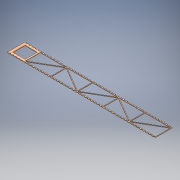
# Autodesk Inventor part: bottom
Saved by Autodesk Inventor 2018.3 (Build 223284000, 284)
## iProperties
Created: 2018-05-24
Part Number: bottom
Material: Wood (Birch)
Document SubType Name: Modeling
Designer: mzhang
Density: 0.55 g/cm^3
Appearance: Birch - Natural Polished
Mass: 4.54021 g
Surface Area: 164.361 cm^2
Volume: 8.25494 cm^3
Author: mzhang
Autodesk Inventor part; units mm, degrees
ref_plane "YZ Plane" through (0, 0, 0) normal (1, 0, 0) x (0, 1, 0)
ref_plane "XZ Plane" through (0, 0, 0) normal (0, 1, 0) x (-1, 0, 0)
ref_plane "XY Plane" through (0, 0, 0) normal (0, 0, 1) x (1, 0, 0)
sketch "Sketch1" plane through (0, 0, 0) normal (0, 0, 1) x (1, 0, 0)
  line L0 (0, 0) -> (40, 0)
  line L1 (40, 0) -> (40, 40)
  line L2 (40, 40) -> (0, 40)
  line L3 (0, 40) -> (0, 0)
  line L4 (45, 40) -> (45, -3.586)
  line L5 (470, 43.586) -> (470, -5)
  line L6 (472.0842, 45.0353) -> (472.0575, -4.9647)
  line L7 (45, 40) -> (45, -3.586)
  line L8 (470, -5) -> (470, 43.586)
  line L9 (45, -3.586) -> (128.586, 45)
  line L10 (46.414, -5) -> (129.078, 43.0501)
  line L11 (129.078, -5) -> (129.078, 43.0501)
  line L12 (131, 43.0501) -> (131, -5)
  line L13 (131, -5) -> (129, 45) construction
  line L14 (129.078, -5) -> (131.078, 45) construction
  line L15 (214, -3.0047) -> (214, 45)
  line L16 (216, 45) -> (216, -3.0047)
  line L17 (299.078, -5) -> (299.078, 43.0501)
  line L18 (301, 43.0501) -> (301, -5)
  line L19 (301, -5) -> (299, 45) construction
  line L20 (299.078, -5) -> (301.078, 45) construction
  line L21 (384.0797, -3.0079) -> (384.0797, 44.9968)
  line L22 (386, 45) -> (386, -3.0501)
  line L23 (386.0782, -5.0063) -> (384.0797, 44.9968) construction
  line L24 (384, -5) -> (386, 45) construction
  line L25 (214, -3.0047) -> (131.414, 45)
  line L26 (213.664, -5) -> (131, 43.0501)
  line L27 (216.414, -5) -> (299.078, 43.0501)
  line L28 (216, -3.0047) -> (298.586, 45)
  line L29 (384.0797, -3.0079) -> (301.4937, 44.9968)
  line L30 (383.664, -5) -> (301, 43.0501)
  line L31 (386, -3.0501) -> (468.586, 45)
  line L32 (386.414, -5) -> (469.078, 43.0501)
  line L33 (469.078, 43.0501) -> (470, 43.586)
  line L34 (-7, 45) -> (40, 45)
  line L35 (0, 45) -> (9, 45)
  line L36 (-7, 45) -> (-7, -5)
  line L37 (-7, -5) -> (40, -5)
  line L38 (40, 45) -> (45, 45)
  line L39 (45, 45) -> (45, 40)
  line L40 (-8.9425, 47.0353) -> (-8.9425, -6.9647)
  line L41 (472.0575, 47.0353) -> (472.0842, 47.0353)
  line L42 (472.0842, 47.0353) -> (472.0842, 45.0353)
  line L43 (472.0575, -4.9647) -> (472.0575, -6.9647)
  line L44 (-8.9425, 47.0353) -> (472.0842, 47.0353)
  line L45 (472.0575, -6.9647) -> (-8.9425, -6.9647)
  line L46 (45, 45) -> (128.586, 45)
  line L47 (131.414, 45) -> (214, 45)
  line L48 (216, 45) -> (298.586, 45)
  line L49 (301.4937, 44.9968) -> (384.0797, 44.9968)
  line L50 (386, 45) -> (468.586, 45)
  line L51 (213.664, -5) -> (131, -5)
  line L52 (40, -5) -> (129.078, -5)
  line L53 (216.414, -5) -> (299.078, -5)
  line L54 (301, -5) -> (383.664, -5)
  line L55 (386.414, -5) -> (470, -5)
  point P0 (20, 20)
  point P1 (385, -3.586)
  point P2 (215, -3.586)
  dimension "d0" = 40
  dimension "d1" = 40
  constraints: 113 end point, 12 parallel, 11 point on line, 6 perpendicular, 4 collinear, 4 horizontal, 2 vertical
  measures "d0" distance of L2.end L1.end
  measures "d1" distance of L1.end L0.end
extrude "Extrusion1" add sketch "Sketch1" along normal blind 1.5875
sketch "Sketch2" plane through (-8.9425, -6.9647, 0) normal (0, -1, 0) x (1, 0, 0)
  line L0 (0, 0) -> (0, 1.5875) projected
  line L1 (481.0267, 1.5875) -> (0, 1.5875) projected
  line L2 (0, 0) -> (5, 0)
  line L3 (5, 0) -> (5, 1.5875)
  line L4 (5, 1.5875) -> (0, 1.5875)
  line L5 (0, 1.5875) -> (0, 0)
  point P0 (8.9425, 0)
  dimension "d64" = 5
  constraints: 8 end point, 2 parallel, 1 horizontal, 1 perpendicular, 1 point on line
  measures "d64" distance of L4.end L3.end
extrude "Extrusion2" add sketch "Sketch2" along normal blind 1.5875
pattern_linear "Rectangular Pattern1" count 48 spacing 10 along (1, 0, 0) of "Extrusion2"
sketch "Sketch3" plane through (-8.9425, 47.0353, 0) normal (0, 1, 0) x (1, 0, 0)
  line L0 (0, 0) -> (481.0267, 0) projected
  line L1 (481.0267, -1.5875) -> (0, -1.5875) projected
  line L2 (0, 0) -> (5, 0)
  line L3 (5, 0) -> (5, -1.5875)
  line L4 (5, -1.5875) -> (0, -1.5875)
  line L5 (0, -1.5875) -> (0, 0)
  point P0 (8.9425, 0)
  dimension "d70" = 5
  constraints: 8 end point, 2 parallel, 1 horizontal, 1 perpendicular, 1 point on line
  measures "d70" distance of L3.end L4.end
extrude "Extrusion3" add sketch "Sketch3" along normal blind 1.5875
pattern_linear "Rectangular Pattern2" count 48 spacing 10 along (1, 0, 0) of "Extrusion3"
sketch "Sketch4" plane through (0, 0, 1.5875) normal (0, 0, 1) x (1, 0, 0)
  line L0 (472.0575, -6.9647) -> (472.0575, -4.9647) projected
  line L1 (472.0575, -6.9647) -> (473.7973, -6.9647)
  line L2 (473.7973, -6.9647) -> (473.7973, 49.231)
  line L3 (473.7973, 49.231) -> (472.0575, 49.231)
  line L4 (472.0575, 49.231) -> (472.0575, -6.9647)
  point P0 (0, 0)
  constraints: 8 end point, 2 parallel, 1 horizontal, 1 perpendicular
extrude "Extrusion4" cut sketch "Sketch4" against normal up to surface (1.5875 mm away)
body "Solid1"
